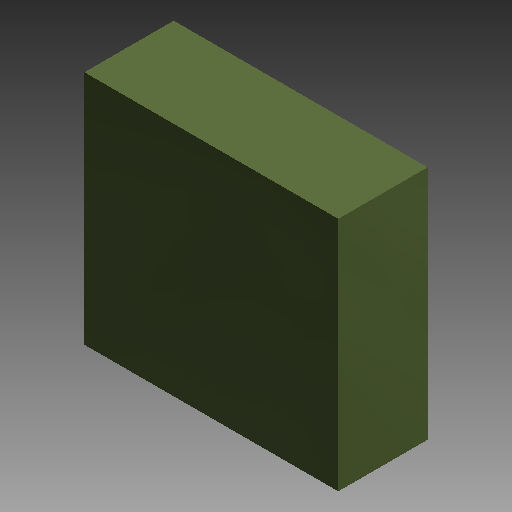
# Autodesk Inventor part: S3A-13-F
Saved by Autodesk Inventor 2018.2 (Build 222227000, 227)
## iProperties
Part Number: S3A-13-F
Material: Generic
Document SubType Name: Modeling
Designer: autocad
Appearance: DO-214AB, S3A-13-F
Author: autocad
Autodesk Inventor part; units mm, degrees
ref_plane "YZ Plane" through (0, 0, 0) normal (1, 0, 0) x (0, 1, 0)
ref_plane "XZ Plane" through (0, 0, 0) normal (0, 1, 0) x (-1, 0, 0)
ref_plane "XY Plane" through (0, 0, 0) normal (0, 0, 1) x (1, 0, 0)
sketch "DO-214AB, S3A-13-F_175" plane through (0, 0, 0) normal (0, 0, 1) x (1, 0, 0)
  line L0 (3.556, 3.302) -> (3.556, -3.3008)
  line L1 (3.556, -3.3008) -> (-3.5508, -3.3008)
  line L2 (-3.5508, -3.3008) -> (-3.5508, 3.302)
  line L3 (-3.5508, 3.302) -> (3.556, 3.302)
  constraints: 8 end point
extrude "Extrusion1" add sketch "DO-214AB, S3A-13-F_175" along normal blind 2.5
body "Solid1"
